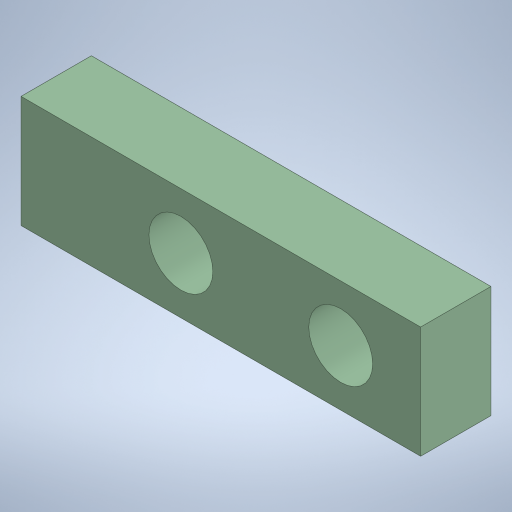
# Autodesk Inventor part: griper_base_TPU
Saved by Autodesk Inventor 2024 (Build 280153000, 153)
## iProperties
Created: 2025-06-02
Part Number: griper_base_TPU
Material: ゴム、シリコーン
Document SubType Name: Modeling
Designer: 1412z
Density: 1.25 g/cm^3
Appearance: ゴム - 緑
Author: 1412z
Autodesk Inventor part; units mm, degrees
ref_plane "YZ Plane" through (0, 0, 0) normal (1, 0, 0) x (0, 1, 0)
ref_plane "XZ Plane" through (0, 0, 0) normal (0, 1, 0) x (-1, 0, 0)
ref_plane "XY Plane" through (0, 0, 0) normal (0, 0, 1) x (1, 0, 0)
sketch "スケッチ1" plane through (0, 0, 0) normal (0, 0, 1) x (1, 0, 0)
  line L0 (12.5, -3.5) -> (-12.5, -3.5)
  line L1 (-12.5, -3.5) -> (-12.5, 3.5)
  line L2 (-12.5, 3.5) -> (12.5, 3.5)
  line L3 (12.5, 3.5) -> (12.5, -3.5)
  line L4 (12.5, -3.5) -> (-12.5, 3.5) construction
  line L5 (-12.5, -3.5) -> (12.5, 3.5) construction
  circle A0 centre (7.5, 0) radius 2
  circle A1 centre (-2.5, 0) radius 2
  point P0 (0, 0)
  dimension "d0" = 25
  dimension "d1" = 7
  dimension "d2" = 4
  dimension "d3" = 4
  constraints: 12 end point, 2 centre point, 2 midpoint, 2 parallel, 1 horizontal, 1 perpendicular
  measures "d0" distance of L1.end L2.end
  measures "d1" distance of L0.end L1.end
  measures "d2" diameter of A0
  measures "d3" diameter of A1
extrude "押し出し1" add sketch "スケッチ1" along normal blind 4.4
